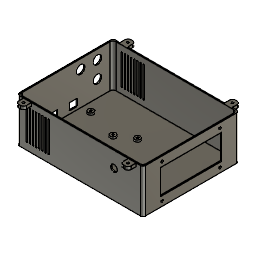
Caixa (Autodesk Fusion 360 design; units mm, degrees)
Autodesk Fusion 360 part; units mm, degrees
note: some values were not read from the file. Set by a fixed rule: which sketch regions a step uses.
other "Recurso de malha base1"
other "Escala1"
other "Modificar1"
other "Modificar2"
sketch "Esboço2" plane through (6.5, 0, 0) normal (1, 0, 0) x (0, 1, 0)
  arc A0 (6.1394, 12.4997) -> (5.5505, 11.9276) centre (6.1499, 11.8998) ccw
  line L0 (5.5505, 11.9276) -> (5.5505, 2.5236)
  arc A1 (5.5505, 2.5236) -> (6.15, 1.9) centre (6.1501, 2.5) ccw
  arc A2 (16.9488, 1.9) -> (17.5486, 2.5005) centre (16.9486, 2.5) ccw
  line L1 (17.5486, 2.5005) -> (17.5486, 11.9396)
  arc A3 (17.5486, 11.9396) -> (16.9471, 12.4997) centre (16.9499, 11.8997) ccw
  line L2 (16.9471, 12.4997) -> (6.1394, 12.4997)
  line L3 (16.9488, 1.9) -> (6.15, 1.9)
  line L4 (-14.125, 12.45) -> (-14.125, 1.6)
  line L5 (-14.125, 1.6) -> (-22.975, 1.6)
  line L6 (-22.975, 1.6) -> (-22.975, 12.45)
  line L7 (-22.975, 12.45) -> (-14.125, 12.45)
  line L8 (5.2505, 11.9339) -> (5.2505, 2.5288)
  arc A4 (5.2505, 2.5288) -> (6.15, 1.6) centre (6.1501, 2.5) ccw
  line L9 (16.9488, 1.6) -> (6.15, 1.6)
  arc A5 (16.9488, 1.6) -> (17.8486, 2.5006) centre (16.9486, 2.5) ccw
  line L10 (17.8486, 2.5006) -> (17.8486, 11.9486)
  arc A6 (17.8486, 11.9486) -> (16.9464, 12.7997) centre (16.9499, 11.8997) ccw
  line L11 (16.9464, 12.7997) -> (6.1371, 12.7997)
  arc A7 (6.1371, 12.7997) -> (5.2505, 11.9339) centre (6.1499, 11.8998) ccw
  line L12 (-13.825, 1.3) -> (-23.275, 1.3)
  line L13 (-23.275, 1.3) -> (-23.275, 12.75)
  line L14 (-23.275, 12.75) -> (-13.825, 12.75)
  line L15 (-13.825, 12.75) -> (-13.825, 1.3)
  dimension "d5" = 0.6
  dimension "d7" = 0.3
  dimension "d8" = -0.3
  constraint vertical L1
  constraint horizontal L2
  constraint vertical L0
  constraint equal A0 A2
  constraint equal A2 A3
  constraint equal A1 A2
  constraint horizontal L3
  constraint vertical L4
  constraint horizontal L7
  constraint vertical L6
  constraint horizontal L5
  measures "d5" radius of A2
other "CorteDeMalha2"
sketch "Esboço3" plane through (0, 0, 0) normal (0, 0, 1) x (1, 0, 0)
  circle A0 centre (21.8, 24.15) radius 1.75
  circle A1 centre (20.5, -24.15) radius 1.75
  circle A2 centre (72.6, -18.95) radius 1.75
  circle A3 centre (72.6, 8.95) radius 1.75
  circle A4 centre (103, -24.15) radius 1.75
  circle A5 centre (96.7, 24.15) radius 1.75
  circle A6 centre (20.5, -24.15) radius 3.5
  circle A7 centre (21.8, 24.15) radius 3.5
  circle A8 centre (72.6, 8.95) radius 3.5
  circle A9 centre (96.7, 24.15) radius 3.5
  circle A10 centre (72.6, -18.95) radius 3.5
  circle A11 centre (103, -24.15) radius 3.5
  circle A12 centre (20.5, -24.15) radius 4.5
  circle A13 centre (21.8, 24.15) radius 4.5
  circle A14 centre (72.6, 8.95) radius 4.5
  circle A15 centre (72.6, -18.95) radius 4.5
  circle A16 centre (103, -24.15) radius 4.5
  circle A17 centre (96.7, 24.15) radius 4.5
  line L0 (6.5, 35.001) -> (6.5, -40)
  dimension "d6" = 3.5
  dimension "d12" = 7
  dimension "d13" = 9
  dimension "d15" = 15.3
  constraint equal A3 A5
  constraint equal A0 A3
  constraint equal A0 A2
  constraint equal A2 A4
  constraint equal A1 A2
  constraint concentric A1 A6
  constraint concentric A0 A7
  constraint concentric A3 A8
  constraint concentric A5 A9
  constraint concentric A2 A10
  constraint concentric A4 A11
  constraint equal A7 A9
  constraint equal A8 A9
  constraint equal A8 A10
  constraint equal A10 A11
  constraint equal A6 A11
  constraint concentric A6 A12
  constraint concentric A0 A13
  constraint concentric A3 A14
  constraint concentric A2 A15
  constraint concentric A11 A16
  constraint concentric A9 A17
  constraint equal A13 A14
  constraint equal A12 A14
  constraint equal A12 A17
  constraint equal A16 A17
  constraint equal A15 A16
  constraint vertical L0
  measures "d6" diameter of A1
  measures "d12" diameter of A6
  measures "d13" diameter of A12
  measures "d15" distance of A0.centre L0
other "CorteDeMalha3"
ref_plane "Plano de trabalho1" through (0, 0, -5) normal (0, 0, 1) x (1, 0, 0)
sketch "Esboço5" plane through (0, 0, -5) normal (0, 0, 1) x (1, 0, 0)
  circle A0 centre (21.8, 24.15) radius 3.5
  circle A1 centre (72.6, 8.95) radius 1.75
  circle A2 centre (20.5, -24.15) radius 1.75
  circle A3 centre (96.7, 24.15) radius 1.75
  circle A4 centre (96.7, 24.15) radius 4.5
  circle A5 centre (103, -24.15) radius 4.5
  circle A6 centre (21.8, 24.15) radius 1.75
  circle A7 centre (72.6, 8.95) radius 4.5
  circle A8 centre (72.6, -18.95) radius 4.5
  circle A9 centre (96.7, 24.15) radius 3.5
  circle A10 centre (20.5, -24.15) radius 3.5
  circle A11 centre (103, -24.15) radius 1.75
  circle A12 centre (20.5, -24.15) radius 4.5
  circle A13 centre (72.6, -18.95) radius 3.5
  circle A14 centre (72.6, 8.95) radius 3.5
  circle A15 centre (21.8, 24.15) radius 4.5
  circle A16 centre (103, -24.15) radius 3.5
  circle A17 centre (72.6, -18.95) radius 1.75
  line L0 (6.5, 75) -> (204.4068, 75)
  line L1 (204.4068, 75) -> (204.4068, -75)
  line L2 (204.4068, -75) -> (6.5, -75)
  line L3 (6.5, -75) -> (6.5, 75)
  line L4 (21.8, 24.15) -> (20.5, -24.15)
  line L5 (38.6076, 75) -> (38.6076, -75)
  line L6 (21.15, 0) -> (38.6076, 0)
  point P0 (21.15, 0)
  point P1 (38.6076, 0)
  dimension "d20" = 3.5
  dimension "d21" = 7
  dimension "d22" = 9
  dimension "d24" = 15.3
  dimension "d25" = 150
  constraint equal A1 A3
  constraint equal A1 A6
  constraint equal A6 A17
  constraint equal A11 A17
  constraint equal A2 A17
  constraint concentric A2 A10
  constraint concentric A0 A6
  constraint concentric A1 A14
  constraint concentric A3 A9
  constraint concentric A13 A17
  constraint concentric A11 A16
  constraint equal A0 A9
  constraint equal A9 A14
  constraint equal A13 A14
  constraint equal A13 A16
  constraint equal A10 A16
  constraint concentric A10 A12
  constraint concentric A6 A15
  constraint concentric A1 A7
  constraint concentric A8 A17
  constraint concentric A5 A16
  constraint concentric A4 A9
  constraint equal A7 A15
  constraint equal A7 A12
  constraint equal A4 A12
  constraint equal A4 A5
  constraint equal A5 A8
  constraint horizontal L0
  constraint vertical L1
  constraint horizontal L2
  constraint vertical L3
  constraint coincident A0.centre A6.centre
  constraint coincident A2.centre A10.centre
  constraint midpoint L4 P0
  constraint coincident L0 L5.start
  constraint coincident L2 L5.end
  constraint perpendicular L2 L5
  constraint midpoint L5 P1
  constraint coincident P0 L6.start
  constraint coincident P1 L6.end
  constraint horizontal L6
  measures "d20" diameter of A2
  measures "d21" diameter of A10
  measures "d22" diameter of A12
  measures "d24" distance of A0.centre L3
  measures "d25" distance of L0 L2
extrude "Extrusão1" add sketch "Esboço5" along normal blind 2 contours L0 L2 L3 L5 | L0 L1 L2 L5 makes body 1
extrude "Extrusão2" add sketch "Esboço5" along normal blind 3.5 contours A4 | A5 | A7 | A8 | A12 | A15 bodies 1
extrude "Extrusão3" add sketch "Esboço3" against normal blind 1.5 contours A6 | A7 | A8 | A9 | A10 | A11 | A12 | A13 | A14 | A15 | A16 | A17 bodies 1
ref_plane "Plano de trabalho3" through (6.5, 0, 0) normal (1, 0, 0) x (0, 1, 0)
sketch "Esboço7" plane through (6.5, 0, 0) normal (1, 0, 0) x (0, 1, 0)
  line L0 (-14.125, 1.6) -> (-22.975, 1.6)
  line L1 (-23.275, 12.75) -> (-13.825, 12.75)
  line L2 (5.2505, 11.9339) -> (5.2505, 2.5288)
  arc A0 (16.9488, 1.6) -> (17.8486, 2.5006) centre (16.9486, 2.5) ccw
  line L3 (-13.825, 1.3) -> (-23.275, 1.3)
  line L4 (-13.825, 12.75) -> (-13.825, 1.3)
  arc A1 (17.8486, 11.9486) -> (16.9464, 12.7997) centre (16.9499, 11.8997) ccw
  line L5 (17.8486, 2.5006) -> (17.8486, 11.9486)
  arc A2 (16.9488, 1.9) -> (17.5486, 2.5005) centre (16.9486, 2.5) ccw
  line L6 (16.9464, 12.7997) -> (6.1371, 12.7997)
  line L7 (-14.125, 12.45) -> (-14.125, 1.6)
  arc A3 (6.1371, 12.7997) -> (5.2505, 11.9339) centre (6.1499, 11.8998) ccw
  line L8 (-22.975, 12.45) -> (-14.125, 12.45)
  line L9 (-22.975, 1.6) -> (-22.975, 12.45)
  line L10 (16.9488, 1.6) -> (6.15, 1.6)
  arc A4 (17.5486, 11.9396) -> (16.9471, 12.4997) centre (16.9499, 11.8997) ccw
  line L11 (16.9488, 1.9) -> (6.15, 1.9)
  line L12 (17.5486, 2.5005) -> (17.5486, 11.9396)
  arc A5 (6.1394, 12.4997) -> (5.5505, 11.9276) centre (6.1499, 11.8998) ccw
  line L13 (5.5505, 11.9276) -> (5.5505, 2.5236)
  line L14 (-23.275, 1.3) -> (-23.275, 12.75)
  line L15 (16.9471, 12.4997) -> (6.1394, 12.4997)
  arc A6 (5.2505, 2.5288) -> (6.15, 1.6) centre (6.1501, 2.5) ccw
  arc A7 (5.5505, 2.5236) -> (6.15, 1.9) centre (6.1501, 2.5) ccw
  line L16 (-75, -3) -> (-75, -5)
  line L17 (-75, -5) -> (75, -5)
  line L18 (75, -5) -> (75, -3)
  line L19 (75, -5) -> (-75, -5)
  line L20 (-75, -5) -> (-75, 65)
  line L21 (-75, 65) -> (75, 65)
  line L22 (75, 65) -> (75, -5)
  circle A8 centre (50, 23.2) radius 6.7
  circle A9 centre (50, 50) radius 6.7
  circle A10 centre (23.2, 50) radius 6.7
  line L23 (50, 50) -> (50, 23.2)
  line L24 (50, 50) -> (23.2, 50)
  dimension "d34" = 0.3
  dimension "d35" = -0.3
  dimension "d36" = 0.6
  dimension "d40" = 70
  dimension "d45" = 13.4
  dimension "d46" = 13.4
  dimension "d47" = 26.8
  dimension "d48" = 13.4
  dimension "d50" = 26.8
  dimension "d72" = 25
  dimension "d73" = 15
  constraint vertical L12
  constraint horizontal L15
  constraint vertical L13
  constraint equal A2 A5
  constraint equal A2 A4
  constraint equal A2 A7
  constraint horizontal L11
  constraint vertical L7
  constraint horizontal L8
  constraint vertical L9
  constraint horizontal L0
  constraint horizontal L19
  constraint vertical L20
  constraint horizontal L21
  constraint vertical L22
  constraint coincident A9.centre L23.start
  constraint coincident A8.centre L23.end
  constraint coincident A10.centre L24.end
  constraint vertical L23
  constraint horizontal L24
  measures "d36" radius of A2
  measures "d40" distance of L17.end L21.end
  measures "d45" diameter of A8
  measures "d46" diameter of A9
  measures "d47" distance of A8.centre A9.centre
  measures "d48" diameter of A10
  measures "d50" distance of A9.centre A10.centre
  measures "d72" distance of L22 A9.centre
  measures "d73" distance of L21 A9.centre
extrude "Extrusão5" add sketch "Esboço7" against normal blind 2 contours L16 L17 L18 L19 L20 L21 L22 bodies 1
ref_plane "Plano de trabalho5" through (104.4534, -75, 30) normal (0, -1, 0) x (1, 0, 0)
sketch "Esboço10" plane through (0, -75, 0) normal (0, -1, 0) x (-1, 0, 0)
  line L0 (-204.4068, 5) -> (-204.4068, 3)
  line L1 (-204.4068, 3) -> (-6.5, 3)
  line L2 (-6.5, 3) -> (-6.5, -65)
  line L3 (-6.5, -65) -> (-4.5, -65)
  line L4 (-4.5, -65) -> (-4.5, 5)
  line L5 (-4.5, 5) -> (-6.5, 5)
  line L6 (-6.5, 5) -> (-204.4068, 5)
  line L7 (-4.5, 5) -> (-204.4068, 5)
  line L8 (-204.4068, 5) -> (-204.4068, -65)
  line L9 (-204.4068, -65) -> (-4.5, -65)
  line L10 (-4.5, -65) -> (-4.5, 5)
  circle A0 centre (-160, -40) radius 5.36
  line L11 (-44.5, -55.0001) -> (-44.5, -6.9999)
  line L12 (-34.5, -55.0001) -> (-34.5, -6.9999)
  arc A1 (-35.4977, -56.0001) -> (-34.5, -55.0001) centre (-35.5, -55.0001) ccw
  arc A2 (-36.5, -55.0001) -> (-35.4977, -56.0001) centre (-35.5, -55.0001) ccw
  arc A3 (-50.4977, -56.0001) -> (-49.5, -55.0001) centre (-50.5, -55.0001) ccw
  line L13 (-51.5, -6.9999) -> (-51.5, -55.0001)
  arc A4 (-55.4977, -56.0001) -> (-54.5, -55.0001) centre (-55.5, -55.0001) ccw
  line L14 (-19.5, -55.0001) -> (-19.5, -6.9999)
  arc A5 (-20.4977, -56.0001) -> (-19.5, -55.0001) centre (-20.5, -55.0001) ccw
  arc A6 (-40.5195, -6.0001) -> (-41.5, -6.9999) centre (-40.5, -6.9999) ccw
  line L15 (-31.5, -6.9999) -> (-31.5, -55.0001)
  arc A7 (-19.5, -6.9999) -> (-20.5195, -6.0001) centre (-20.5, -6.9999) ccw
  arc A8 (-51.5, -55.0001) -> (-50.4977, -56.0001) centre (-50.5, -55.0001) ccw
  arc A9 (-25.5195, -6.0001) -> (-26.5, -6.9999) centre (-25.5, -6.9999) ccw
  arc A10 (-26.5, -55.0001) -> (-25.4977, -56.0001) centre (-25.5, -55.0001) ccw
  arc A11 (-40.4977, -56.0001) -> (-39.5, -55.0001) centre (-40.5, -55.0001) ccw
  arc A12 (-34.5, -6.9999) -> (-35.5195, -6.0001) centre (-35.5, -6.9999) ccw
  arc A13 (-45.4977, -56.0001) -> (-44.5, -55.0001) centre (-45.5, -55.0001) ccw
  arc A14 (-45.5195, -6.0001) -> (-46.5, -6.9999) centre (-45.5, -6.9999) ccw
  line L16 (-46.5, -6.9999) -> (-46.5, -55.0001)
  line L17 (-29.5, -55.0001) -> (-29.5, -6.9999)
  arc A15 (-21.5, -55.0001) -> (-20.4977, -56.0001) centre (-20.5, -55.0001) ccw
  arc A16 (-30.4977, -56.0001) -> (-29.5, -55.0001) centre (-30.5, -55.0001) ccw
  arc A17 (-46.5, -55.0001) -> (-45.4977, -56.0001) centre (-45.5, -55.0001) ccw
  arc A18 (-31.5, -55.0001) -> (-30.4977, -56.0001) centre (-30.5, -55.0001) ccw
  arc A19 (-56.5, -55.0001) -> (-55.4977, -56.0001) centre (-55.5, -55.0001) ccw
  line L18 (-21.5, -6.9999) -> (-21.5, -55.0001)
  arc A20 (-41.5, -55.0001) -> (-40.4977, -56.0001) centre (-40.5, -55.0001) ccw
  line L19 (-55.5, -55.0001) -> (-55.5, -6.9999)
  line L20 (-24.5, -55.0001) -> (-24.5, -6.9999)
  arc A21 (-54.5, -6.9999) -> (-55.5195, -6.0001) centre (-55.5, -6.9999) ccw
  arc A22 (-39.5, -6.9999) -> (-40.5195, -6.0001) centre (-40.5, -6.9999) ccw
  arc A23 (-35.5195, -6.0001) -> (-36.5, -6.9999) centre (-35.5, -6.9999) ccw
  line L21 (-26.5, -6.9999) -> (-26.5, -55.0001)
  line L22 (-56.5, -6.9999) -> (-56.5, -55.0001)
  arc A24 (-25.4977, -56.0001) -> (-24.5, -55.0001) centre (-25.5, -55.0001) ccw
  arc A25 (-44.5, -6.9999) -> (-45.5195, -6.0001) centre (-45.5, -6.9999) ccw
  arc A26 (-30.5195, -6.0001) -> (-31.5, -6.9999) centre (-30.5, -6.9999) ccw
  arc A27 (-24.5, -6.9999) -> (-25.5195, -6.0001) centre (-25.5, -6.9999) ccw
  line L23 (-36.5, -6.9999) -> (-36.5, -55.0001)
  line L24 (-54.5, -55.0001) -> (-54.5, -6.9999)
  arc A28 (-29.5, -6.9999) -> (-30.5195, -6.0001) centre (-30.5, -6.9999) ccw
  line L25 (-49.5, -55.0001) -> (-49.5, -6.9999)
  arc A29 (-55.5195, -6.0001) -> (-56.5, -6.9999) centre (-55.5, -6.9999) ccw
  line L26 (-41.5, -6.9999) -> (-41.5, -55.0001)
  arc A30 (-49.5, -6.9999) -> (-50.5195, -6.0001) centre (-50.5, -6.9999) ccw
  line L27 (-39.5, -55.0001) -> (-39.5, -6.9999)
  arc A31 (-20.5195, -6.0001) -> (-21.5, -6.9999) centre (-20.5, -6.9999) ccw
  arc A32 (-50.5195, -6.0001) -> (-51.5, -6.9999) centre (-50.5, -6.9999) ccw
  line L28 (-85, 3) -> (-85, -65)
  line L29 (-85, -31) -> (-55.5, -31)
  point P0 (-55.5, -31)
  point P1 (-55.5, -31)
  point P2 (-85, -31)
  dimension "d74" = 10.72
  dimension "d85" = 35
  dimension "d86" = 0
  dimension "d87" = 2
  dimension "d88" = 1
  dimension "d89" = 1
  dimension "d90" = 13
  dimension "d128" = 50
  constraint horizontal L7
  constraint vertical L8
  constraint horizontal L9
  constraint vertical L10
  constraint coincident L4.end L5.start
  constraint coincident L3.end L4.start
  constraint coincident L0.start L6.end
  constraint vertical L24
  constraint vertical L22
  constraint tangent A4 L24
  constraint tangent A19 L22
  constraint equal A4 A19
  constraint coincident A4.start A19.end
  constraint tangent A21 L24
  constraint tangent L22 A29
  constraint equal A21 A29
  constraint coincident A21.end A29.start
  constraint coincident A4.centre A19.centre
  constraint coincident L19.end A21.centre
  constraint midpoint P1 L19
  constraint coincident P1 P0
  constraint coincident L1 L28.start
  constraint perpendicular L1 L28
  constraint coincident L9 L28.end
  constraint midpoint L28 P2
  constraint coincident P2 L29.start
  constraint horizontal L29
  measures "d74" diameter of A0
  measures "d87" distance of L22 L24
  measures "d88" radius of A4
  measures "d89" radius of A21
  measures "d90" distance of L2 L14
  measures "d128" vertical distance of A5.start A7.end
extrude "Extrusão6" add sketch "Esboço10" along normal blind 2 bodies 1
ref_plane "Plano de trabalho6" through (104.4534, 75, 30) normal (0, 1, 0) x (-1, 0, 0)
sketch "Esboço11" plane through (0, 75, 0) normal (0, 1, 0) x (1, 0, 0)
  line L0 (204.4068, 3) -> (204.4068, 5)
  line L1 (204.4068, 5) -> (4.5, 5)
  line L2 (4.5, 5) -> (4.5, -65)
  line L3 (4.5, -65) -> (6.5, -65)
  line L4 (6.5, -65) -> (6.5, 3)
  line L5 (6.5, 3) -> (204.4068, 3)
  line L6 (4.5, 5) -> (204.4068, 5)
  line L7 (204.4068, 5) -> (204.4068, -65)
  line L8 (204.4068, -65) -> (4.5, -65)
  line L9 (4.5, -65) -> (4.5, 5)
  line L10 (21.5, -55.0001) -> (21.5, -6.9999)
  line L11 (19.5, -6.9999) -> (19.5, -55.0001)
  arc A0 (20.5023, -56.0001) -> (21.5, -55.0001) centre (20.5, -55.0001) ccw
  arc A1 (19.5, -55.0001) -> (20.5023, -56.0001) centre (20.5, -55.0001) ccw
  arc A2 (21.5, -6.9999) -> (20.4805, -6.0001) centre (20.5, -6.9999) ccw
  arc A3 (20.4805, -6.0001) -> (19.5, -6.9999) centre (20.5, -6.9999) ccw
  line L12 (61.469, -65) -> (61.469, 3)
  line L13 (20.5, -55.0001) -> (20.5, -6.9999)
  line L14 (61.469, -31) -> (20.5, -31)
  line L15 (26.5, -55.0001) -> (26.5, -6.9999)
  arc A4 (26.5, -6.9999) -> (25.4805, -6.0001) centre (25.5, -6.9999) ccw
  arc A5 (25.4805, -6.0001) -> (24.5, -6.9999) centre (25.5, -6.9999) ccw
  line L16 (24.5, -6.9999) -> (24.5, -55.0001)
  arc A6 (24.5, -55.0001) -> (25.5023, -56.0001) centre (25.5, -55.0001) ccw
  arc A7 (25.5023, -56.0001) -> (26.5, -55.0001) centre (25.5, -55.0001) ccw
  line L17 (31.5, -55.0001) -> (31.5, -6.9999)
  arc A8 (31.5, -6.9999) -> (30.4805, -6.0001) centre (30.5, -6.9999) ccw
  arc A9 (30.4805, -6.0001) -> (29.5, -6.9999) centre (30.5, -6.9999) ccw
  line L18 (29.5, -6.9999) -> (29.5, -55.0001)
  arc A10 (29.5, -55.0001) -> (30.5023, -56.0001) centre (30.5, -55.0001) ccw
  arc A11 (30.5023, -56.0001) -> (31.5, -55.0001) centre (30.5, -55.0001) ccw
  line L19 (36.5, -55.0001) -> (36.5, -6.9999)
  arc A12 (36.5, -6.9999) -> (35.4805, -6.0001) centre (35.5, -6.9999) ccw
  arc A13 (35.4805, -6.0001) -> (34.5, -6.9999) centre (35.5, -6.9999) ccw
  line L20 (34.5, -6.9999) -> (34.5, -55.0001)
  arc A14 (34.5, -55.0001) -> (35.5023, -56.0001) centre (35.5, -55.0001) ccw
  arc A15 (35.5023, -56.0001) -> (36.5, -55.0001) centre (35.5, -55.0001) ccw
  line L21 (41.5, -55.0001) -> (41.5, -6.9999)
  arc A16 (41.5, -6.9999) -> (40.4805, -6.0001) centre (40.5, -6.9999) ccw
  arc A17 (40.4805, -6.0001) -> (39.5, -6.9999) centre (40.5, -6.9999) ccw
  line L22 (39.5, -6.9999) -> (39.5, -55.0001)
  arc A18 (39.5, -55.0001) -> (40.5023, -56.0001) centre (40.5, -55.0001) ccw
  arc A19 (40.5023, -56.0001) -> (41.5, -55.0001) centre (40.5, -55.0001) ccw
  line L23 (46.5, -55.0001) -> (46.5, -6.9999)
  arc A20 (46.5, -6.9999) -> (45.4805, -6.0001) centre (45.5, -6.9999) ccw
  arc A21 (45.4805, -6.0001) -> (44.5, -6.9999) centre (45.5, -6.9999) ccw
  line L24 (44.5, -6.9999) -> (44.5, -55.0001)
  arc A22 (44.5, -55.0001) -> (45.5023, -56.0001) centre (45.5, -55.0001) ccw
  arc A23 (45.5023, -56.0001) -> (46.5, -55.0001) centre (45.5, -55.0001) ccw
  line L25 (51.5, -55.0001) -> (51.5, -6.9999)
  arc A24 (51.5, -6.9999) -> (50.4805, -6.0001) centre (50.5, -6.9999) ccw
  arc A25 (50.4805, -6.0001) -> (49.5, -6.9999) centre (50.5, -6.9999) ccw
  line L26 (49.5, -6.9999) -> (49.5, -55.0001)
  arc A26 (49.5, -55.0001) -> (50.5023, -56.0001) centre (50.5, -55.0001) ccw
  arc A27 (50.5023, -56.0001) -> (51.5, -55.0001) centre (50.5, -55.0001) ccw
  line L27 (56.5, -55.0001) -> (56.5, -6.9999)
  arc A28 (56.5, -6.9999) -> (55.4805, -6.0001) centre (55.5, -6.9999) ccw
  arc A29 (55.4805, -6.0001) -> (54.5, -6.9999) centre (55.5, -6.9999) ccw
  line L28 (54.5, -6.9999) -> (54.5, -55.0001)
  arc A30 (54.5, -55.0001) -> (55.5023, -56.0001) centre (55.5, -55.0001) ccw
  arc A31 (55.5023, -56.0001) -> (56.5, -55.0001) centre (55.5, -55.0001) ccw
  point P0 (61.469, -31)
  point P1 (20.5, -31)
  dimension "d75" = 2
  dimension "d76" = 1
  dimension "d77" = 1
  dimension "d80" = 35
  dimension "d81" = 0
  dimension "d82" = 13
  dimension "d129" = 50
  constraint horizontal L6
  constraint vertical L7
  constraint horizontal L8
  constraint vertical L9
  constraint coincident L1.end L2.start
  constraint coincident L2.end L3.start
  constraint coincident L0.end L1.start
  constraint vertical L10
  constraint vertical L11
  constraint tangent L10 A0
  constraint tangent L11 A1
  constraint equal A0 A1
  constraint coincident A0.start A1.end
  constraint tangent L10 A2
  constraint tangent L11 A3
  constraint equal A2 A3
  constraint coincident A2.end A3.start
  constraint coincident L8 L12.start
  constraint coincident L5 L12.end
  constraint perpendicular L5 L12
  constraint midpoint L12 P0
  constraint coincident A0.centre A1.centre
  constraint coincident A2.centre A3.centre
  constraint midpoint L13 P1
  constraint coincident P0 L14.start
  constraint coincident P1 L14.end
  constraint horizontal L14
  measures "d75" distance of L10 L11
  measures "d76" radius of A0
  measures "d77" radius of A2
  measures "d82" distance of L4 L11
  measures "d129" vertical distance of A0.start A2.end
extrude "Extrusão7" add sketch "Esboço11" along normal blind 2 bodies 1
ref_plane "Plano de trabalho7" through (204.4068, 0, 30) normal (1, 0, 0) x (0, 1, 0)
sketch "Esboço12" plane through (204.4068, 0, 0) normal (1, 0, 0) x (0, 1, 0)
  line L0 (-77, -5) -> (-75, -5)
  line L1 (-75, -5) -> (77, -5)
  line L2 (77, -5) -> (77, 65)
  line L3 (77, 65) -> (75, 65)
  line L4 (75, 65) -> (75, -3)
  line L5 (75, -3) -> (-75, -3)
  line L6 (-75, -3) -> (-75, 65)
  line L7 (-75, 65) -> (-77, 65)
  line L8 (-77, 65) -> (-77, -5)
  line L9 (-77, -5) -> (77, -5)
  line L10 (77, -5) -> (77, 65)
  line L11 (77, 65) -> (-77, 65)
  line L12 (-77, 65) -> (-77, -5)
  line L13 (49, 9.9) -> (49, 50.1)
  line L14 (49, 50.1) -> (-49, 50.1)
  line L15 (-49, 50.1) -> (-49, 9.9)
  line L16 (-49, 9.9) -> (49, 9.9)
  circle A0 centre (-46.3, 2.7) radius 1.95
  circle A1 centre (46.3, 2.7) radius 1.95
  circle A2 centre (46.3, 57.3) radius 1.95
  circle A3 centre (-46.3, 57.3) radius 1.95
  line L17 (-49, 50.1) -> (49, 9.9)
  line L18 (-46.3, 57.3) -> (46.3, 2.7)
  line L19 (-77, 65) -> (77, -5)
  dimension "d57" = 98
  dimension "d58" = 40.2
  dimension "d59" = 3.9
  dimension "d60" = 3.9
  dimension "d61" = 92.6
  dimension "d62" = 3.9
  dimension "d63" = 3.9
  dimension "d64" = 92.6
  dimension "d65" = 54.6
  constraint horizontal L9
  constraint vertical L10
  constraint horizontal L11
  constraint vertical L12
  constraint coincident L2.end L3.start
  constraint coincident L0.start L8.end
  constraint horizontal L16
  constraint vertical L13
  constraint horizontal L14
  constraint vertical L15
  constraint horizontal A3.centre A2.centre
  constraint horizontal A0.centre A1.centre
  constraint vertical A3.centre A0.centre
  constraint coincident A3.centre L18.start
  constraint coincident A1.centre L18.end
  constraint midpoint L17 L18
  constraint coincident L7.end L8.start
  constraint coincident L1.end L2.start
  constraint midpoint L17 L19
  measures "d57" distance of L15.end L13.start
  measures "d58" distance of L15.end L14.end
  measures "d59" diameter of A3
  measures "d60" diameter of A2
  measures "d61" horizontal distance of A3.centre A2.centre
  measures "d62" diameter of A0
  measures "d63" diameter of A1
  measures "d64" horizontal distance of A0.centre A1.centre
  measures "d65" vertical distance of A3.centre A0.centre
extrude "Extrusão8" add sketch "Esboço12" along normal blind 2 contours L0 L1 L5 L6 L8 L9 L12 L19 | L6 L7 L11 L19 | L2 L3 L4 L5 L10 L11 L19 | L4 L5 L6 L11 L13 L14 L16 L19 | L5 L6 L14 L15 L16 L19 bodies 1
fillet "Arredondamento1" radius 5 4 edges at (204.4068, -75, 31) (204.4068, 75, 31) (6.5, 75, 31) (6.5, -75, 31) on bodies 1
fillet "Arredondamento2" radius 4 4 edges at (206.4068, 77, 30) (206.4068, -77, 30) (4.5, 77, 30) (4.5, -77, 30) on bodies 1
ref_plane "Plano de trabalho8" through (105.4534, 0, 65) normal (0, 0, 1) x (0, 1, 0)
sketch "Esboço13" plane through (0, 0, 65) normal (0, 0, 1) x (1, 0, 0)
  arc A0 (11.5, -75) -> (6.5, -70) centre (11.5, -70) cw
  line L0 (6.5, -70) -> (6.5, 70)
  arc A1 (6.5, 70) -> (11.5, 75) centre (11.5, 70) cw
  line L1 (11.5, 75) -> (199.4068, 75)
  arc A2 (199.4068, 75) -> (204.4068, 70) centre (199.4068, 70) cw
  line L2 (204.4068, 70) -> (204.4068, -70)
  arc A3 (204.4068, -70) -> (199.4068, -75) centre (199.4068, -70) cw
  line L3 (199.4068, -75) -> (11.5, -75)
  line L4 (11.5, -75) -> (6.5, -75)
  line L5 (6.5, -75) -> (6.5, -70)
  line L6 (204.4068, -70) -> (204.4068, -75)
  line L7 (204.4068, -75) -> (199.4068, -75)
  line L8 (6.5, -75) -> (5.0359, -75)
  arc A4 (5.0359, -75) -> (8.5, -77) centre (8.5, -73) ccw
  line L9 (8.5, -77) -> (202.4068, -77)
  arc A5 (202.4068, -77) -> (204.4068, -76.4641) centre (202.4068, -73) ccw
  arc A6 (204.4068, -76.4641) -> (206.4068, -73) centre (202.4068, -73) ccw
  line L10 (206.4068, -73) -> (206.4068, 73)
  arc A7 (206.4068, 73) -> (202.4068, 77) centre (202.4068, 73) ccw
  line L11 (202.4068, 77) -> (8.5, 77)
  arc A8 (8.5, 77) -> (4.5, 73) centre (8.5, 73) ccw
  line L12 (4.5, 73) -> (4.5, -73)
  arc A9 (4.5, -73) -> (5.0359, -75) centre (8.5, -73) ccw
  line L13 (204.4068, -75) -> (204.4068, -76.4641)
  line L14 (24.9401, -81.5801) -> (21.7401, -79.7326)
  line L15 (21.7401, -79.7326) -> (18.5401, -81.5801)
  line L16 (18.5401, -81.5801) -> (18.5401, -85.2751)
  line L17 (18.5401, -85.2751) -> (21.7401, -87.1227)
  line L18 (21.7401, -87.1227) -> (24.9401, -85.2751)
  line L19 (24.9401, -85.2751) -> (24.9401, -81.5801)
  circle A10 centre (21.7401, -83.4276) radius 1.75
  line L20 (15.5, -77) -> (27.9802, -77)
  line L21 (27.9802, -77) -> (27.9802, -84.8553)
  line L22 (22.9802, -89.8553) -> (20.5, -89.8553)
  line L23 (15.5, -84.8553) -> (15.5, -77)
  arc A11 (15.5, -84.8553) -> (20.5, -89.8553) centre (20.5, -84.8553) ccw
  arc A12 (22.9802, -89.8553) -> (27.9802, -84.8553) centre (22.9802, -84.8553) ccw
  line L24 (195.4068, -77) -> (195.4068, -84.8553)
  arc A13 (190.4068, -89.8553) -> (195.4068, -84.8553) centre (190.4068, -84.8553) ccw
  line L25 (190.4068, -89.8553) -> (187.9266, -89.8553)
  arc A14 (182.9266, -84.8553) -> (187.9266, -89.8553) centre (187.9266, -84.8553) ccw
  line L26 (182.9266, -84.8553) -> (182.9266, -77)
  line L27 (182.9266, -77) -> (195.4068, -77)
  line L28 (189.1667, -87.1227) -> (192.3667, -85.2752)
  line L29 (192.3667, -85.2752) -> (192.3667, -81.5801)
  line L30 (192.3667, -81.5801) -> (189.1667, -79.7326)
  line L31 (189.1667, -79.7326) -> (185.9667, -81.5801)
  line L32 (185.9667, -85.2752) -> (189.1667, -87.1227)
  line L33 (185.9667, -81.5801) -> (185.9667, -85.2752)
  circle A15 centre (189.1667, -83.4276) radius 1.75
  arc A16 (190.4068, -89.8553) -> (195.4068, -84.8553) centre (190.4068, -84.8553) ccw
  line L34 (190.4068, -89.8553) -> (187.9266, -89.8553)
  arc A17 (182.9266, -84.8553) -> (187.9266, -89.8553) centre (187.9266, -84.8553) ccw
  line L35 (182.9266, -84.8553) -> (182.9266, -77)
  line L36 (182.9266, -77) -> (195.4068, -77)
  line L37 (195.4068, -77) -> (195.4068, -84.8553)
  line L38 (189.1667, -79.7326) -> (185.9667, -81.5801)
  line L39 (185.9667, -81.5801) -> (185.9667, -85.2752)
  line L40 (185.9667, -85.2752) -> (189.1667, -87.1227)
  line L41 (189.1667, -87.1227) -> (192.3667, -85.2752)
  line L42 (192.3667, -81.5801) -> (189.1667, -79.7326)
  line L43 (192.3667, -85.2752) -> (192.3667, -81.5801)
  circle A18 centre (189.1667, -83.4276) radius 1.75
  arc A19 (187.9266, 89.8552) -> (182.9266, 84.8552) centre (187.9266, 84.8552) ccw
  line L44 (187.9266, 89.8552) -> (190.4068, 89.8552)
  arc A20 (195.4068, 84.8552) -> (190.4068, 89.8552) centre (190.4068, 84.8552) ccw
  line L45 (195.4068, 84.8552) -> (195.4068, 77)
  line L46 (195.4068, 77) -> (182.9266, 77)
  line L47 (182.9266, 77) -> (182.9266, 84.8552)
  line L48 (189.1667, 79.7326) -> (192.3667, 81.5801)
  line L49 (192.3667, 81.5801) -> (192.3667, 85.2751)
  line L50 (192.3667, 85.2751) -> (189.1667, 87.1227)
  line L51 (189.1667, 87.1227) -> (185.9667, 85.2751)
  line L52 (185.9667, 81.5801) -> (189.1667, 79.7326)
  line L53 (185.9667, 85.2751) -> (185.9667, 81.5801)
  circle A21 centre (189.1667, 83.4276) radius 1.75
  arc A22 (20.5, 89.8552) -> (15.5, 84.8552) centre (20.5, 84.8552) ccw
  line L54 (20.5, 89.8552) -> (22.9802, 89.8552)
  arc A23 (27.9802, 84.8552) -> (22.9802, 89.8552) centre (22.9802, 84.8552) ccw
  line L55 (27.9802, 84.8552) -> (27.9802, 77)
  line L56 (27.9802, 77) -> (15.5, 77)
  line L57 (15.5, 77) -> (15.5, 84.8552)
  line L58 (21.7401, 79.7326) -> (24.9401, 81.5801)
  line L59 (24.9401, 81.5801) -> (24.9401, 85.2751)
  line L60 (24.9401, 85.2751) -> (21.7401, 87.1227)
  line L61 (21.7401, 87.1227) -> (18.5401, 85.2751)
  line L62 (18.5401, 81.5801) -> (21.7401, 79.7326)
  line L63 (18.5401, 85.2751) -> (18.5401, 81.5801)
  circle A24 centre (21.7401, 83.4276) radius 1.75
  point P0 (21.7401, -83.4276)
  point P1 (21.7401, -83.4276)
  dimension "d98" = 3.2
  dimension "d99" = 3.5
  dimension "d101" = 11
  dimension "d102" = 5
  dimension "d103" = 3.5
  dimension "d104" = 5
  dimension "d105" = 6.2401
  dimension "d106" = 3.0401
  dimension "d107" = 11
  dimension "d110" = 3.5
  dimension "d111" = 5
  dimension "d112" = 6.2401
  dimension "d113" = 3.0401
  dimension "d114" = 3.5
  dimension "d115" = 5
  dimension "d116" = 6.2401
  dimension "d117" = 3.0401
  dimension "d118" = 11
  dimension "d119" = 3.5
  dimension "d120" = 5
  dimension "d121" = 6.2401
  dimension "d122" = 3.0401
  dimension "d123" = 11
  dimension "d136" = 0
  dimension "d137" = 0
  constraint coincident P1 P0
  constraint vertical L16
  constraint horizontal L20
  constraint vertical L21
  constraint horizontal L22
  constraint vertical L23
  constraint coincident L9 L20.start
  constraint tangent L22 A11
  constraint tangent L23 A11
  constraint tangent L21 A12
  constraint tangent L22 A12
  constraint equal A11 A12
  constraint vertical L33
  constraint horizontal L27
  constraint vertical L24
  constraint horizontal L25
  constraint vertical L26
  constraint tangent L25 A14
  constraint tangent A14 L26
  constraint tangent L24 A13
  constraint tangent A13 L25
  constraint equal A13 A14
  constraint coincident L9 L24.start
  constraint vertical L39
  constraint horizontal L36
  constraint vertical L37
  constraint horizontal L34
  constraint vertical L35
  constraint tangent L34 A17
  constraint tangent A17 L35
  constraint tangent A16 L37
  constraint tangent A16 L34
  constraint equal A16 A17
  constraint tangent L44 A20
  constraint tangent A20 L45
  constraint tangent A19 L47
  constraint tangent A19 L44
  constraint equal A19 A20
  constraint coincident L11 L46.end
  constraint tangent L54 A23
  constraint tangent A23 L55
  constraint tangent A22 L57
  constraint tangent A22 L54
  constraint equal A22 A23
  constraint coincident L11 L55.end
  measures "d98" distance of P1 L19
  measures "d99" diameter of A10
  measures "d101" distance of L12 L23
  measures "d102" radius of A11
  measures "d103" diameter of A15
  measures "d104" radius of A14
  measures "d105" distance of A15.centre L26
  measures "d106" distance of L26 L33
  measures "d107" distance of L10 L24
  measures "d110" diameter of A18
  measures "d111" radius of A17
  measures "d112" distance of A15.centre L35
  measures "d113" distance of L35 L39
  measures "d114" diameter of A21
  measures "d115" radius of A20
  measures "d116" distance of A21.centre L45
  measures "d117" distance of L45 L49
  measures "d118" distance of L10 L45
  measures "d119" diameter of A24
  measures "d120" radius of A23
  measures "d121" distance of A24.centre L55
  measures "d122" distance of L55 L59
  measures "d123" distance of L12 L57
extrude "Extrusão9" add sketch "Esboço13" against normal blind 2 contours L9 L20 L21 L22 L23 A11 A12 | L14 L15 L16 L17 L18 L19 bodies 1
extrude "Extrusão10" add sketch "Esboço13" against normal blind 5 contours L9 L20 L21 L22 L23 A11 A12 bodies 1
extrude "Extrusão11" add sketch "Esboço13" against normal blind 2 contours L9 L24 A13 L25 A14 L26 L27 A16 L34 A17 L35 L36 L37 | L11 A22 L54 A23 L55 L56 L57 | L11 A19 L44 A20 L45 L46 L47 | L28 L29 L30 L31 L32 L33 L38 L39 L40 L41 L42 L43 | L48 L49 L50 L51 L52 L53 | L58 L59 L60 L61 L62 L63 bodies 1
extrude "Extrusão12" add sketch "Esboço13" against normal blind 5 contours L9 L24 A13 L25 A14 L26 L27 A16 L34 A17 L35 L36 L37 | L11 A22 L54 A23 L55 L56 L57 | L11 A19 L44 A20 L45 L46 L47 bodies 1
sketch "Esboço14" plane through (0, 0, 0) normal (0, 0, 1) x (1, 0, 0)
  line L0 (8.5, -77) -> (202.4068, -77)
  line L1 (204.4068, -70) -> (204.4068, -75)
  line L2 (206.4068, -73) -> (206.4068, 73)
  arc A0 (204.4068, -70) -> (199.4068, -75) centre (199.4068, -70) cw
  line L3 (190.4068, -89.8553) -> (187.9266, -89.8553)
  line L4 (190.4068, -89.8553) -> (187.9266, -89.8553)
  arc A1 (190.4068, -89.8553) -> (195.4068, -84.8553) centre (190.4068, -84.8553) ccw
  line L5 (182.9266, -77) -> (195.4068, -77)
  line L6 (182.9266, -77) -> (195.4068, -77)
  line L7 (4.5, 73) -> (4.5, -73)
  circle A2 centre (189.1667, -83.4276) radius 1.75
  line L8 (6.5, -70) -> (6.5, 70)
  arc A3 (187.9266, 89.8552) -> (182.9266, 84.8552) centre (187.9266, 84.8552) ccw
  line L9 (182.9266, 77) -> (182.9266, 84.8552)
  arc A4 (195.4068, 84.8552) -> (190.4068, 89.8552) centre (190.4068, 84.8552) ccw
  line L10 (11.5, 75) -> (199.4068, 75)
  arc A5 (199.4068, 75) -> (204.4068, 70) centre (199.4068, 70) cw
  line L11 (195.4068, 77) -> (182.9266, 77)
  arc A6 (15.5, -84.8553) -> (20.5, -89.8553) centre (20.5, -84.8553) ccw
  arc A7 (11.5, -75) -> (6.5, -70) centre (11.5, -70) cw
  line L12 (22.9802, -89.8553) -> (20.5, -89.8553)
  line L13 (6.5, -75) -> (5.0359, -75)
  line L14 (15.5, -77) -> (27.9802, -77)
  line L15 (6.5, -75) -> (6.5, -70)
  line L16 (27.9802, -77) -> (27.9802, -84.8553)
  line L17 (187.9266, 89.8552) -> (190.4068, 89.8552)
  line L18 (195.4068, 84.8552) -> (195.4068, 77)
  line L19 (204.4068, 70) -> (204.4068, -70)
  line L20 (202.4068, 77) -> (8.5, 77)
  circle A8 centre (189.1667, 83.4276) radius 1.75
  arc A9 (206.4068, 73) -> (202.4068, 77) centre (202.4068, 73) ccw
  line L21 (199.4068, -75) -> (11.5, -75)
  line L22 (15.5, 77) -> (15.5, 84.8552)
  arc A10 (6.5, 70) -> (11.5, 75) centre (11.5, 70) cw
  line L23 (27.9802, 84.8552) -> (27.9802, 77)
  arc A11 (190.4068, -89.8553) -> (195.4068, -84.8553) centre (190.4068, -84.8553) ccw
  line L24 (204.4068, -75) -> (204.4068, -76.4641)
  line L25 (15.5, -84.8553) -> (15.5, -77)
  arc A12 (20.5, 89.8552) -> (15.5, 84.8552) centre (20.5, 84.8552) ccw
  arc A13 (4.5, -73) -> (5.0359, -75) centre (8.5, -73) ccw
  line L26 (20.5, 89.8552) -> (22.9802, 89.8552)
  line L27 (27.9802, 77) -> (15.5, 77)
  line L28 (195.4068, -77) -> (195.4068, -84.8553)
  line L29 (182.9266, -84.8553) -> (182.9266, -77)
  arc A14 (182.9266, -84.8553) -> (187.9266, -89.8553) centre (187.9266, -84.8553) ccw
  circle A15 centre (189.1667, -83.4276) radius 1.75
  line L30 (204.4068, -75) -> (199.4068, -75)
  arc A16 (202.4068, -77) -> (204.4068, -76.4641) centre (202.4068, -73) ccw
  arc A17 (8.5, 77) -> (4.5, 73) centre (8.5, 73) ccw
  line L31 (195.4068, -77) -> (195.4068, -84.8553)
  arc A18 (204.4068, -76.4641) -> (206.4068, -73) centre (202.4068, -73) ccw
  arc A19 (22.9802, -89.8553) -> (27.9802, -84.8553) centre (22.9802, -84.8553) ccw
  circle A20 centre (21.7401, 83.4276) radius 1.75
  circle A21 centre (21.7401, -83.4276) radius 1.75
  arc A22 (27.9802, 84.8552) -> (22.9802, 89.8552) centre (22.9802, 84.8552) ccw
  line L32 (11.5, -75) -> (6.5, -75)
  line L33 (182.9266, -84.8553) -> (182.9266, -77)
  arc A23 (5.0359, -75) -> (8.5, -77) centre (8.5, -73) ccw
  arc A24 (182.9266, -84.8553) -> (187.9266, -89.8553) centre (187.9266, -84.8553) ccw
  circle A25 centre (189.1667, -83.4276) radius 3.5
  circle A26 centre (21.7401, -83.4276) radius 3.5
  circle A27 centre (21.7401, 83.4276) radius 3.5
  circle A28 centre (189.1667, 83.4276) radius 3.5
  point P0 (21.7401, -83.4276)
  point P1 (21.7401, -83.4276)
  dimension "d143" = 3.5
  dimension "d144" = 11
  dimension "d145" = 5
  dimension "d146" = 3.5
  dimension "d147" = 5
  dimension "d148" = 6.2401
  dimension "d150" = 11
  dimension "d151" = 3.5
  dimension "d152" = 5
  dimension "d153" = 6.2401
  dimension "d155" = 3.5
  dimension "d156" = 5
  dimension "d157" = 6.2401
  dimension "d159" = 11
  dimension "d160" = 3.5
  dimension "d161" = 5
  dimension "d162" = 6.2401
  dimension "d164" = 11
  dimension "d165" = 7
  dimension "d166" = 7
  dimension "d167" = 7
  dimension "d168" = 7
  constraint coincident P1 P0
  constraint horizontal L14
  constraint vertical L16
  constraint horizontal L12
  constraint vertical L25
  constraint coincident L14.start L0
  constraint tangent A6 L12
  constraint tangent A6 L25
  constraint tangent L16 A19
  constraint tangent L12 A19
  constraint equal A6 A19
  constraint horizontal L5
  constraint vertical L31
  constraint horizontal L4
  constraint vertical L29
  constraint tangent L4 A14
  constraint tangent L29 A14
  constraint tangent A1 L31
  constraint tangent L4 A1
  constraint equal A1 A14
  constraint coincident L5.end L0
  constraint horizontal L6
  constraint vertical L28
  constraint horizontal L3
  constraint vertical L33
  constraint tangent L3 A24
  constraint tangent L33 A24
  constraint tangent A11 L28
  constraint tangent L3 A11
  constraint equal A11 A24
  constraint tangent A4 L17
  constraint tangent A4 L18
  constraint tangent A3 L9
  constraint tangent A3 L17
  constraint equal A3 A4
  constraint coincident L9.start L20
  constraint tangent L26 A22
  constraint tangent L23 A22
  constraint tangent L22 A12
  constraint tangent A12 L26
  constraint equal A12 A22
  constraint coincident L23.end L20
  constraint concentric A15 A25
  constraint concentric A20 A27
  constraint concentric A8 A28
  measures "d143" diameter of A21
  measures "d144" distance of L7 L25
  measures "d145" radius of A6
  measures "d146" diameter of A15
  measures "d147" radius of A14
  measures "d148" distance of A2.centre L29
  measures "d150" distance of L2 L31
  measures "d151" diameter of A2
  measures "d152" radius of A24
  measures "d153" distance of A2.centre L33
  measures "d155" diameter of A8
  measures "d156" radius of A4
  measures "d157" distance of A8.centre L18
  measures "d159" distance of L2 L18
  measures "d160" diameter of A20
  measures "d161" radius of A22
  measures "d162" distance of A20.centre L23
  measures "d164" distance of L7 L22
  measures "d165" diameter of A25
  measures "d166" diameter of A26
  measures "d167" diameter of A27
  measures "d168" diameter of A28
extrude "Extrusão13" add sketch "Esboço14" along normal blind 2 separate body contours L0 L5 L6 L13 L14 L21 L24 L30 A16 L32 A23 | L1 L2 L7 L8 L10 A5 L11 L13 L15 L19 L20 A9 A10 L24 A13 L27 A17 A18 | A7 L15 L32 | A0 L8 L10 A5 A7 L19 L21 A10 | L1 A0 L30 makes body 2
extrude "Extrusão14" add sketch "Esboço14" along normal blind 3.5 contours L0 A6 L12 L14 L16 L25 A19 | L0 L3 L4 A1 L5 L6 A11 L28 L29 A14 L31 L33 A24 | L20 L22 L23 A12 L26 L27 A22 | A3 L9 A4 L11 L17 L18 L20 bodies 2
chamfer "Chanfro1" distance 1.5 angle 45 4 edges at (189.1667, 77, 3.5) (21.7401, 77, 3.5) (189.1667, -77, 3.5) (21.7401, -77, 3.5) on bodies 2
sketch "Esboço15" plane through (0, 0, 2) normal (0, 0, 1) x (-1, 0, 0)
  arc A0 (-4.5, 73) -> (-8.5, 77) centre (-8.5, 73) ccw
  line L0 (-8.5, 77) -> (-15.5, 77)
  line L1 (-15.5, 77) -> (-27.9802, 77)
  line L2 (-27.9802, 77) -> (-182.9266, 77)
  line L3 (-182.9266, 77) -> (-195.4068, 77)
  line L4 (-195.4068, 77) -> (-202.4068, 77)
  arc A1 (-202.4068, 77) -> (-204.4068, 76.4641) centre (-202.4068, 73) ccw
  arc A2 (-204.4068, 76.4641) -> (-206.4068, 73) centre (-202.4068, 73) ccw
  line L5 (-206.4068, 73) -> (-206.4068, -73)
  arc A3 (-206.4068, -73) -> (-202.4068, -77) centre (-202.4068, -73) ccw
  line L6 (-202.4068, -77) -> (-195.4068, -77)
  line L7 (-195.4068, -77) -> (-182.9266, -77)
  line L8 (-182.9266, -77) -> (-27.9802, -77)
  line L9 (-27.9802, -77) -> (-15.5, -77)
  line L10 (-15.5, -77) -> (-8.5, -77)
  arc A4 (-8.5, -77) -> (-4.5, -73) centre (-8.5, -73) ccw
  line L11 (-4.5, -73) -> (-4.5, 73)
  line L12 (-155.9075, 30.1886) -> (-155.9075, -30.1886) construction
  line L13 (-155.9075, -30.1886) -> (-135.5134, -30.1886) construction
  line L14 (-135.5134, -30.1886) -> (-135.5134, 30.1886) construction
  line L15 (-135.5134, 30.1886) -> (-155.9075, 30.1886) construction
  line L16 (-135.5134, 77) -> (-135.5134, -77)
  dimension "d174" = 15
  dimension "d175" = 0
  text T0 "V0.7" font "Arial" height 15 align centre middle in box 60.3773 x 20.3941 at (-155.9075, 30.1886) x (0, -1) y (1, 0) spacing 1
  constraint coincident L2 L16.start
  constraint perpendicular L2 L16
  constraint coincident L8 L16.end
  constraint midpoint L16
extrude "Extrusão15" cut sketch "Esboço15" against normal blind 0.5 text T0 bodies 2
hidden bodies 2
equation "d6 = rArd"
equation "rArd = 3.5 mm"
equation "d12 = 2 * rArd"
equation "d13 = 2 * rArd + 2 mm"
equation "d20 = rArd"
equation "d21 = 2 * rArd"
equation "d22 = 2 * rArd + 2 mm"
equation "d28 = 2 mm + 1.5 mm"
equation "rCoax = 13.4 mm"
equation "d45 = rCoax"
equation "d46 = rCoax"
equation "d47 = 2 * rCoax"
equation "d48 = rCoax"
equation "d50 = 2 * rCoax"
equation "d74 = 0.8 * rCoax"
equation "d99 = rArd"
equation "d103 = rArd"
equation "d110 = rArd"
equation "d114 = rArd"
equation "d119 = rArd"
equation "d143 = rArd"
equation "d146 = rArd"
equation "d151 = rArd"
equation "d155 = rArd"
equation "d160 = rArd"
equation "d165 = 2 * rArd"
equation "d166 = 2 * rArd"
equation "d167 = 2 * rArd"
equation "d168 = 2 * rArd"
equation "d175 = 'V0.7'"
named bodies: "Corpo_Caixa"
